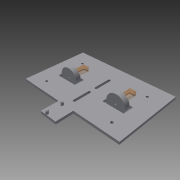
# Autodesk Inventor part: Top
Saved by Autodesk Inventor 2015 (Build 190159000, 159)
## iProperties
Created: 2018-12-21
Part Number: Top
Material: Типовые
Document SubType Name: Modeling
Designer: kostya
Density: 1 g/cm^3
Appearance: По умолчанию
Author: kostya
Autodesk Inventor part; units mm, degrees
ref_plane "YZ Plane" through (0, 0, 0) normal (1, 0, 0) x (0, 1, 0)
ref_plane "XZ Plane" through (0, 0, 0) normal (0, 1, 0) x (-1, 0, 0)
ref_plane "XY Plane" through (0, 0, 0) normal (0, 0, 1) x (1, 0, 0)
sketch "Эскиз1" plane through (0, 0, 0) normal (0, 0, 1) x (1, 0, 0)
  line L0 (-100, -75) -> (100, -75)
  line L1 (100, -75) -> (100, 75)
  line L2 (100, 75) -> (-100, 75)
  line L3 (-100, 75) -> (-100, -75)
  line L4 (-100, -75) -> (100, 75) construction
  line L5 (100, -75) -> (-100, 75) construction
  point P0 (0, 0)
  dimension "d0" = 200
  dimension "d1" = 150
  constraints: 12 end point, 2 midpoint, 2 parallel, 1 horizontal, 1 perpendicular
  measures "d0" distance of L2.end L1.end
  measures "d1" distance of L1.end L0.end
extrude "Выдавливание1" add sketch "Эскиз1" along normal blind 5
sketch "Эскиз2" plane through (0, 0, 5) normal (0, 0, 1) x (1, 0, 0)
  line L0 (100, -75) -> (100, 75) construction
  line L1 (100, 0) -> (-100, 0) construction
  line L2 (-100, 75) -> (-100, -75) construction
  line L3 (100, 75) -> (-100, 75) construction
  line L4 (0, 75) -> (0, -75) construction
  line L5 (-100, -75) -> (100, -75) construction
  line L6 (-100, -10) -> (100, -10) construction
  line L7 (100, -10) -> (100, 10) construction
  line L8 (100, 10) -> (-100, 10) construction
  line L9 (-100, 10) -> (-100, -10) construction
  line L10 (-100, -10) -> (100, 10) construction
  line L11 (100, -10) -> (-100, 10) construction
  line L12 (0, 0) -> (-100, 0) construction
  line L13 (-50, 0) -> (-50, 75) construction
  line L14 (0, 0) -> (100, 0) construction
  line L15 (50, 0) -> (50, 75) construction
  line L16 (-56, 10) -> (-56, 35)
  line L17 (-56, 35) -> (-44, 35)
  line L18 (-44, 35) -> (-44, 10)
  line L19 (-56, 10) -> (-44, 10)
  line L20 (56, 10) -> (56, 35)
  line L21 (56, 35) -> (44, 35)
  line L22 (44, 35) -> (44, 10)
  line L23 (56, 10) -> (44, 10)
  line L24 (-70, -10) -> (-30, -10)
  line L25 (-30, -10) -> (-30, 10)
  line L26 (-30, 10) -> (-70, 10)
  line L27 (-70, 10) -> (-70, -10)
  line L28 (-70, -10) -> (-30, 10) construction
  line L29 (-30, -10) -> (-70, 10) construction
  line L30 (70, -10) -> (30, -10)
  line L31 (30, -10) -> (30, 10)
  line L32 (30, 10) -> (70, 10)
  line L33 (70, 10) -> (70, -10)
  dimension "d4" = 20
  dimension "d7" = 25
  dimension "d8" = 40
  constraints: 60 end point, 10 midpoint, 8 symmetric about line, 7 perpendicular, 6 point on line, 4 parallel, 2 collinear, 2 horizontal, 1 vertical
  measures "d4" distance of L7.end L6.end
  measures "d7" distance of L16.start L16.end
  measures "d8" distance of L26.end L25.end
extrude "Выдавливание2" cut sketch "Эскиз2" against normal blind 2 contours L16 L17 L18 L19 | L23 L22 L21 L20
extrude "Выдавливание3" cut sketch "Эскиз2" against normal blind 5 contours L19 L26 L25 L24 L27 | L32 L33 L30 L31 L23
sketch "Эскиз3" plane through (0, 0, 3) normal (0, 0, 1) x (1, 0, 0)
  line L0 (-56, 10) -> (-56, 35) projected
  line L1 (-44, 10) -> (-56, 10) projected
  line L2 (-44, 35) -> (-44, 10) projected
  line L3 (-56, 35) -> (-44, 35) projected
  line L4 (-44, 35) -> (-44, 10) projected
  point P0 (0, 0)
surface extrude "ВыдавПврх1" sketch "Эскиз3" along normal blind 10 shown yes curves L4 L1 L0 L3
boundary_patch "Участок поверхности1"
sketch "Эскиз4" plane through (-56, 10, 3) normal (0, -1, 0) x (1, 0, 0)
  line L0 (0, 10) -> (12, 10) construction
  line L1 (6, 10) -> (6, 0) construction
  line L2 (12, 0) -> (0, 0) construction
  line L3 (0, 0) -> (0, 10) construction
  line L4 (0, 5) -> (12, 5) construction
  line L5 (12, 0) -> (12, 10) construction
  arc A0 (7.118, 4) -> (4.882, 4) centre (6, 5) ccw
  line L6 (6, 3.5) -> (6, 4) construction
  line L7 (6, 4) -> (7.118, 4)
  line L8 (6, 4) -> (4.882, 4)
  point P0 (56, -3)
  dimension "d17" = 3
  dimension "d18" = 0.5
  constraints: 10 end point, 5 midpoint, 2 point on circle, 2 point on line, 1 centre point, 1 horizontal, 1 perpendicular
  measures "d17" diameter of A0
  measures "d18" distance of L6.start L6.end
surface extrude "ВыдавПврх2" sketch "Эскиз4" along normal blind 10 shown yes curves L7 A0 L8
boundary_patch "Участок поверхности2"
mirror "Зеркальное отражение1" about plane through (0, 0, 0) normal (1, 0, 0) of "ВыдавПврх1", "ВыдавПврх2"
ref_plane "РабПлоскость1" through (-70, 0, 5) normal (0, -1, 0) x (1, 0, 0)
sketch "Эскиз5" plane through (-70, 0, 5) normal (0, -1, 0) x (1, 0, 0)
  arc A0 (21.118, 2) -> (18.882, 2) centre (20, 3) ccw projected
  line L0 (18.882, 2) -> (21.118, 2) projected
  circle A1 centre (20, 3) radius 17.5
  point P0 (70, -5)
  dimension "d23" = 35
  constraints: 1 centre point, 1 coincident
  measures "d23" diameter of A1
extrude "Выдавливание4" add sketch "Эскиз5" along normal mid plane 10
mirror "Зеркальное отражение2" about plane through (0, 0, 0) normal (1, 0, 0) of "Выдавливание4"
sketch "Эскиз6" plane through (0, 0, 5) normal (0, 0, 1) x (1, 0, 0)
  line L0 (-100, -75) -> (100, -75) projected
  line L1 (100, -75) -> (100, 75) projected
  line L2 (100, 75) -> (-100, 75) projected
  line L3 (-100, 75) -> (-100, -75) projected
  line L4 (-44, 10) -> (-30, 10) projected
  line L5 (-30, 10) -> (-30, -10) projected
  line L6 (-30, -10) -> (-70, -10) projected
  line L7 (-70, -10) -> (-70, 10) projected
  line L8 (-70, 10) -> (-56, 10) projected
  line L9 (-56, 10) -> (-56, 35) projected
  line L10 (-56, 35) -> (-44, 35) projected
  line L11 (-44, 35) -> (-44, 10) projected
  line L12 (30, 10) -> (44, 10) projected
  line L13 (44, 10) -> (44, 35) projected
  line L14 (44, 35) -> (56, 35) projected
  line L15 (56, 35) -> (56, 10) projected
  line L16 (56, 10) -> (70, 10) projected
  line L17 (70, 10) -> (70, -10) projected
  line L18 (70, -10) -> (30, -10) projected
  line L19 (30, -10) -> (30, 10) projected
  line L20 (100, -75) -> (70, -75)
  line L21 (100, -45) -> (100, -75)
  line L22 (-100, 0) -> (100, 0) construction
  line L23 (100, 75) -> (-100, 75) construction
  line L24 (0, 75) -> (0, -75) construction
  circle A0 centre (70, 45) radius 2.5
  line L25 (70, 45) -> (70, 75) construction
  line L26 (70, 45) -> (100, 45) construction
  line L27 (100, -75) -> (100, 75) projected
  line L28 (100, 10) -> (70, 10) construction
  line L29 (70, 10) -> (70, -10) construction
  line L30 (70, -10) -> (100, -10) construction
  line L31 (100, -10) -> (100, 10) construction
  line L32 (70, -75) -> (70, -35) construction
  line L33 (70, -75) -> (110, -75) construction
  line L34 (70, -35) -> (100, -35) construction
  circle A1 centre (70, -35) radius 2.5
  circle A2 centre (-70, 45) radius 2.5
  line L35 (-70, 45) -> (-70, 75) construction
  line L36 (-70, 45) -> (-100, 45) construction
  line L37 (-70, -75) -> (-70, -35) construction
  line L38 (-70, -35) -> (-100, -35) construction
  circle A3 centre (-70, -35) radius 2.5
  line L39 (100, -75) -> (100, -55)
  line L40 (100, -55) -> (-100, -55)
  point P0 (0, 0)
  dimension "d39" = 30
  dimension "d40" = 30
  dimension "d41" = 40
  dimension "d42" = 90
  dimension "d43" = 5
  dimension "d44" = 20
  constraints: 38 end point, 8 symmetric about line, 6 point on line, 4 centre point, 4 coincident, 4 midpoint, 4 perpendicular, 3 horizontal, 2 parallel, 1 vertical, 2 other
  measures "d39" distance of L25.start L25.end
  measures "d40" distance of L25.start L26.end
  measures "d41" distance of L20.end L32.end
  measures "d42" angle of L33 L32
  measures "d43" diameter of A1
  measures "d44" distance of L0.end L39.end
extrude "Выдавливание5" cut sketch "Эскиз6" against normal blind 10 contours A0 | A1 | A2 | A3
sketch "Эскиз7" plane through (0, 0, 5) normal (0, 0, 1) x (1, 0, 0)
  line L0 (-100, -75) -> (100, -75) projected
  line L1 (100, -75) -> (100, 75) projected
  line L2 (100, 75) -> (-100, 75) projected
  line L3 (-100, 75) -> (-100, -75) projected
  line L4 (-44, 10) -> (-30, 10) projected
  line L5 (-30, 10) -> (-30, -10) projected
  line L6 (-30, -10) -> (-70, -10) projected
  line L7 (-70, -10) -> (-70, 10) projected
  line L8 (-70, 10) -> (-56, 10) projected
  line L9 (-56, 10) -> (-56, 35) projected
  line L10 (-56, 35) -> (-44, 35) projected
  line L11 (-44, 35) -> (-44, 10) projected
  line L12 (30, 10) -> (44, 10) projected
  line L13 (44, 10) -> (44, 35) projected
  line L14 (44, 35) -> (56, 35) projected
  line L15 (56, 35) -> (56, 10) projected
  line L16 (56, 10) -> (70, 10) projected
  line L17 (70, 10) -> (70, -10) projected
  line L18 (70, -10) -> (30, -10) projected
  line L19 (30, -10) -> (30, 10) projected
  line L20 (100, 75) -> (-100, 75) construction
  line L21 (-30, 10) -> (30, 10) construction
  line L22 (30, 10) -> (30, 75) construction
  line L23 (30, 75) -> (-30, 75) construction
  line L24 (-30, 75) -> (-30, 10) construction
  line L25 (-100, -75) -> (100, -75) construction
  line L26 (-30, -10) -> (30, -10) construction
  line L27 (30, -10) -> (30, -75) construction
  line L28 (30, -75) -> (-30, -75) construction
  line L29 (-30, -75) -> (-30, -10) construction
  line L30 (100, -75) -> (100, 75) construction
  line L31 (100, -7.5) -> (100, 7.5) construction
  line L32 (100, 7.5) -> (-100, 7.5) construction
  line L33 (-100, 7.5) -> (-100, -7.5) construction
  line L34 (-100, -7.5) -> (100, 7.5) construction
  line L35 (100, -7.5) -> (-100, 7.5) construction
  line L36 (-100, -7.5) -> (-2.5, -7.5) construction
  line L37 (2.5, -7.5) -> (100, -7.5) construction
  line L38 (-100, 75) -> (-100, -75) construction
  line L39 (-100, 0) -> (100, 0) construction
  arc A0 (-2.5, 7.5) -> (2.5, 7.5) centre (0, 7.5) ccw
  line L40 (2.5, 7.5) -> (2.5, 38.1)
  line L41 (-2.5, 38.1) -> (-2.5, 7.5)
  arc A1 (2.5, 38.1) -> (-2.5, 38.1) centre (0, 38.1) ccw
  line L42 (-2.5, 38.1) -> (-2.5, 7.5)
  line L43 (2.5, 7.5) -> (2.5, 38.1)
  line L44 (-2.5, -38.1) -> (-2.5, -7.5)
  line L45 (2.5, -7.5) -> (2.5, -38.1)
  arc A2 (-2.5, -38.1) -> (2.5, -38.1) centre (0, -38.1) ccw
  arc A3 (2.5, -7.5) -> (-2.5, -7.5) centre (0, -7.5) ccw
  point P0 (0, 0)
  dimension "d31" = 15
  constraints: 44 end point, 8 parallel, 8 point on circle, 6 symmetric about line, 4 centre point, 4 horizontal, 4 midpoint, 4 perpendicular, 4 point on line, 1 collinear, 1 other
  measures "d31" distance of L31.end L31.start
extrude "Выдавливание7" cut sketch "Эскиз7" against normal blind 10 contours L41 A1 L40 A0 | L44 A3 L45 A2
extrude "Выдавливание8" cut sketch "Эскиз6" against normal blind 10 contours L3 L40 L1 L0
sketch "Эскиз9" plane through (0, 0, 5) normal (0, 0, 1) x (1, 0, 0)
  line L0 (30, 10) -> (44, 10) projected
  line L1 (44, 10) -> (44, 35) projected
  line L2 (44, 35) -> (56, 35) projected
  line L3 (56, 35) -> (56, 10) projected
  line L4 (56, 10) -> (70, 10) projected
  line L5 (70, 10) -> (70, -10) projected
  line L6 (70, -10) -> (30, -10) projected
  line L7 (30, -10) -> (30, 10) projected
  line L8 (-44, 10) -> (-30, 10) projected
  line L9 (-30, 10) -> (-30, -10) projected
  line L10 (-30, -10) -> (-70, -10) projected
  line L11 (-70, -10) -> (-70, 10) projected
  line L12 (-70, 10) -> (-56, 10) projected
  line L13 (-56, 10) -> (-56, 35) projected
  line L14 (-56, 35) -> (-44, 35) projected
  line L15 (-44, 35) -> (-44, 10) projected
  line L16 (-100, -55) -> (100, -55) projected
  line L17 (100, -55) -> (100, 75) projected
  line L18 (100, 75) -> (-100, 75) projected
  line L19 (-100, 75) -> (-100, -55) projected
  circle A0 centre (-70, -35) radius 2.5 projected
  circle A1 centre (70, -35) radius 2.5 projected
  circle A2 centre (70, 45) radius 2.5 projected
  circle A3 centre (-70, 45) radius 2.5 projected
  arc A4 (2.5, -7.5) -> (-2.5, -7.5) centre (0, -7.5) ccw projected
  line L20 (2.5, -7.5) -> (2.5, -38.1) projected
  arc A5 (-2.5, -38.1) -> (2.5, -38.1) centre (0, -38.1) ccw projected
  line L21 (-2.5, -38.1) -> (-2.5, -7.5) projected
  arc A6 (-2.5, 7.5) -> (2.5, 7.5) centre (0, 7.5) ccw projected
  line L22 (-2.5, 7.5) -> (-2.5, 38.1) projected
  arc A7 (2.5, 38.1) -> (-2.5, 38.1) centre (0, 38.1) ccw projected
  line L23 (2.5, 38.1) -> (2.5, 7.5) projected
  line L24 (0, 75) -> (0, -55) construction
  line L25 (0, -55) -> (16, -55) construction
  line L26 (-100, -55) -> (100, -55) construction
  line L27 (0, -55) -> (-16, -55) construction
  line L28 (-16, -55) -> (16, -55)
  line L29 (16, -55) -> (16, -87)
  line L30 (16, -87) -> (-16, -87)
  line L31 (-16, -87) -> (-16, -55)
  point P0 (0, 0)
  dimension "d47" = 16
  dimension "d48" = 16
  dimension "d49" = 32
  dimension "d50" = 32
  constraints: 14 end point, 2 midpoint, 2 parallel, 2 point on line, 1 horizontal, 1 perpendicular
  measures "d47" distance of L24.end L25.end
  measures "d48" distance of L24.end L27.end
  measures "d49" distance of L29.end L30.end
  measures "d50" distance of L28.end L29.end
extrude "Выдавливание9" add sketch "Эскиз9" against normal up to surface (5 mm away) contours L16 L29 L30 L31
sketch "Эскиз11" plane through (0, 0, 5) normal (0, 0, 1) x (1, 0, 0)
  line L0 (30, 10) -> (44, 10) projected
  line L1 (44, 10) -> (44, 35) projected
  line L2 (44, 35) -> (56, 35) projected
  line L3 (56, 35) -> (56, 10) projected
  line L4 (56, 10) -> (70, 10) projected
  line L5 (70, 10) -> (70, -10) projected
  line L6 (70, -10) -> (30, -10) projected
  line L7 (30, -10) -> (30, 10) projected
  line L8 (-44, 10) -> (-30, 10) projected
  line L9 (-30, 10) -> (-30, -10) projected
  line L10 (-30, -10) -> (-70, -10) projected
  line L11 (-70, -10) -> (-70, 10) projected
  line L12 (-70, 10) -> (-56, 10) projected
  line L13 (-56, 10) -> (-56, 35) projected
  line L14 (-56, 35) -> (-44, 35) projected
  line L15 (-44, 35) -> (-44, 10) projected
  line L16 (-100, -55) -> (-16, -55) projected
  line L17 (-16, -87) -> (-16, -55) projected
  line L18 (16, -87) -> (-16, -87) projected
  line L19 (16, -55) -> (16, -87) projected
  line L20 (16, -55) -> (100, -55) projected
  line L21 (100, -55) -> (100, 75) projected
  line L22 (100, 75) -> (-100, 75) projected
  line L23 (-100, 75) -> (-100, -55) projected
  circle A0 centre (-70, -35) radius 2.5 projected
  circle A1 centre (70, -35) radius 2.5 projected
  circle A2 centre (70, 45) radius 2.5 projected
  circle A3 centre (-70, 45) radius 2.5 projected
  arc A4 (2.5, -7.5) -> (-2.5, -7.5) centre (0, -7.5) ccw projected
  line L24 (2.5, -7.5) -> (2.5, -38.1) projected
  arc A5 (-2.5, -38.1) -> (2.5, -38.1) centre (0, -38.1) ccw projected
  line L25 (-2.5, -38.1) -> (-2.5, -7.5) projected
  arc A6 (-2.5, 7.5) -> (2.5, 7.5) centre (0, 7.5) ccw projected
  line L26 (-2.5, 7.5) -> (-2.5, 38.1) projected
  arc A7 (2.5, 38.1) -> (-2.5, 38.1) centre (0, 38.1) ccw projected
  line L27 (2.5, 38.1) -> (2.5, 7.5) projected
  line L28 (-16, -87) -> (-7.7, -87) construction
  line L29 (-7.7, -87) -> (-5.3, -87)
  line L30 (16, -87) -> (-16, -87) construction
  line L31 (-7.7, -87) -> (-7.7, -82.6) construction
  line L32 (-5.3, -87) -> (-5.3, -82.6) construction
  line L33 (-5.3, -82.6) -> (10, -82.6) construction
  line L34 (10, -82.6) -> (10, -60.2) construction
  line L35 (10, -60.2) -> (-5.3, -60.2) construction
  line L36 (-5.3, -60.2) -> (-5.3, -55.8) construction
  line L37 (-5.3, -55.8) -> (-7.7, -55.8) construction
  line L38 (-7.7, -55.8) -> (-7.7, -60.2) construction
  line L39 (-7.7, -60.2) -> (-12, -60.2) construction
  line L40 (-12, -60.2) -> (-12, -82.6) construction
  line L41 (-12, -82.6) -> (-7.7, -82.6) construction
  line L42 (-5.3, -87) -> (-2.9, -87)
  line L43 (-2.9, -87) -> (-2.9, -83)
  line L44 (-2.9, -83) -> (-5.3, -83)
  line L45 (-5.3, -83) -> (-5.3, -87)
  line L46 (-12, -71.4) -> (10, -71.4) construction
  point P0 (0, 0)
  dimension "d53" = 8.3
  dimension "d54" = 2.4
  dimension "d55" = 4.4
  dimension "d56" = 15.3
  dimension "d57" = 22.4
  dimension "d58" = 4.4
  dimension "d59" = 4.3
  dimension "d60" = 2.4
  dimension "d61" = 4
  constraints: 36 end point, 6 perpendicular, 4 vertical, 3 horizontal, 2 midpoint, 2 parallel, 2 point on line
  measures "d53" distance of L17.start L28.end
  measures "d54" distance of L28.end L29.end
  measures "d55" distance of L28.end L31.end
  measures "d56" distance of L32.end L33.end
  measures "d57" distance of L33.end L34.end
  measures "d58" distance of L35.end L36.end
  measures "d59" distance of L38.end L39.end
  measures "d60" distance of L44.end L43.end
  measures "d61" distance of L43.end L42.end
extrude "Выдавливание10" add sketch "Эскиз11" along normal blind 7 contours L45 L44 L43 L18
sketch "Эскиз12" plane through (-5.3, -87, 5) normal (-1, 0, 0) x (0, 0, 1)
  line L0 (0, 0) -> (0, 4) projected
  line L1 (0, 0) -> (7, 0) projected
  line L2 (7, 4) -> (7, 0) projected
  line L3 (0, 4) -> (7, 4) projected
  line L4 (0, 0) -> (5.5, 0) construction
  line L5 (5.5, 0) -> (5.5, 1.81)
  line L6 (5.5, 0) -> (6.5, 0)
  line L7 (0, 0) -> (7, 0) projected
  line L8 (6.5, 0) -> (6.5, 1.81)
  line L9 (6.5, 1.81) -> (6, 2.2999) construction
  arc A0 (6.5, 1.81) -> (5.5, 1.81) centre (6, 2.2999) ccw
  point P0 (-5, 87)
  dimension "d64" = 5.5
  dimension "d65" = 1.81
  dimension "d66" = 1
  dimension "d67" = 0.7
  constraints: 10 end point, 2 point on circle, 2 point on line, 2 vertical, 1 centre point, 1 coincident
  measures "d64" distance of L0.start L4.end
  measures "d65" distance of L4.end L5.end
  measures "d66" distance of L4.end L6.end
  measures "d67" distance of L8.end L9.end
extrude "Выдавливание11" cut sketch "Эскиз12" against normal blind 7 contours L5 A0 L8 L1
ref_plane "РабПлоскость4" through (-16, -71.4, 0) normal (0, -1, 0) x (1, 0, 0)
ref_plane "РабПлоскость3" through (-7.7, -55.8, 5) normal (0, 1, 0) x (-1, 0, 0)
mirror "Зеркальное отражение3" about plane through (-16, -71.4, 0) normal (0, -1, 0) of "Выдавливание10", "Выдавливание11"
body "SRF1"
body "SRF2"
body "SRF3"
body "SRF4"
body "SRF5"
body "SRF6"
body "SRF7"
